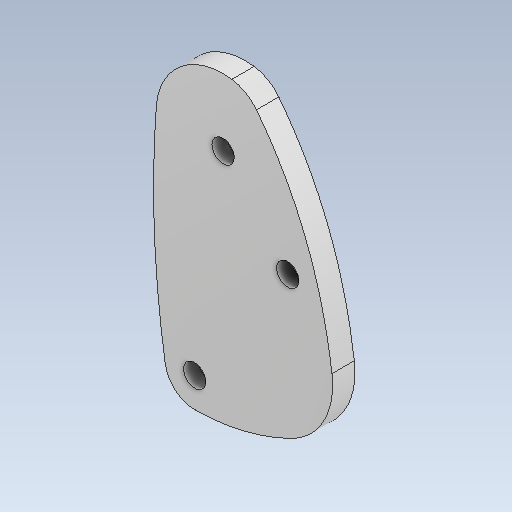
# Autodesk Inventor part: アンノーン後
Saved by Autodesk Inventor 2020.4 (Build 244396000, 396)
## iProperties
Created: 2021-02-23
Part Number: アンノーン後
Material: アルミニウム 2014-T4
Document SubType Name: Modeling
Designer: AA19065
Density: 2.8 g/cm^3
Appearance: サテン
Mass: 6.17685 g
Surface Area: 19.5398 cm^2
Volume: 2.20602 cm^3
Author: AA19065
Autodesk Inventor part; units mm, degrees
ref_plane "YZ Plane" through (0, 0, 0) normal (1, 0, 0) x (0, 1, 0)
ref_plane "XZ Plane" through (0, 0, 0) normal (0, 1, 0) x (-1, 0, 0)
ref_plane "XY Plane" through (0, 0, 0) normal (0, 0, 1) x (1, 0, 0)
sketch "スケッチ1" plane through (0, 0, 0) normal (0, 0, 1) x (1, 0, 0)
  line L0 (108, 72.831817) -> (108, -27.637331) construction
  circle A0 centre (90, 27) radius 3
  circle A1 centre (104.07345, 2) radius 6.025
  circle A2 centre (90, 27) radius 1.5
  circle A3 centre (104.07345, 2) radius 1.5
  circle A4 centre (82.04031, 11.281864) radius 1.5
  circle A5 centre (82.5, -8) radius 3
  circle A6 centre (82.5, -8) radius 1.5
  arc A7 (66.645247, -5.64) -> (72.915941, -4.36) centre (69.780594, -5) ccw
  arc A8 (72.724551, 23.828571) -> (66.645247, -5.64) centre (104.07345, 2) ccw
  arc A9 (77.976723, 20.171429) -> (72.915941, -4.36) centre (104.07345, 2) ccw
  arc A10 (77.976723, 20.171429) -> (72.724551, 23.828571) centre (75.350637, 22) ccw
  circle A11 centre (137.322151, 20) radius 1.25
  circle A12 centre (133.5, -8) radius 3
  circle A13 centre (133.5, -8) radius 1.5
  circle A14 centre (146, 10) radius 1.5
  arc A15 (-6.089587, 13.373015) -> (73.990447, 1.93301) centre (42.288654, 66.020578) ccw construction
  line L1 (108, 72.831817) -> (108, -27.637331) construction
  arc A16 (142.009553, 1.93301) -> (222.089587, 13.373015) centre (173.711346, 66.020578) ccw construction
  arc A17 (142.29705, -19.072921) -> (142.660887, 27.253552) centre (125.709293, 4.222021) ccw
  arc A18 (136.80781, 35.127338) -> (180.06622, 10.718677) centre (180.861669, 62.665248) ccw
  circle A19 centre (137.322151, 20) radius 9.006449
  arc A20 (128.322651, 20.353731) -> (130.555913, -8.5765) centre (253.226204, 15.444317) ccw
  arc A21 (133.414591, -10.998784) -> (152.948723, -4.485529) centre (134.268683, 18.989056) ccw
  arc A22 (35.93378, 10.718677) -> (79.19219, 35.127338) centre (35.138331, 62.665248) ccw
  arc A23 (73.339113, 27.253552) -> (73.70295, -19.072921) centre (90.290707, 4.222021) ccw
  arc A24 (90.887703, 29.865656) -> (71.118535, 25.188537) centre (84.969685, 10.761283) ccw
  arc A25 (109.559222, 4.491371) -> (92.075879, 29.165808) centre (36.719095, -28.589074) ccw
  arc A26 (80.567193, -10.294397) -> (70.653319, -16.566942) centre (76.603177, -15) ccw
  circle A27 centre (76.603177, -15) radius 5 construction
  circle A28 centre (94, -11) radius 1.5
  circle A29 centre (94, -11) radius 3
  arc A30 (103.111347, -3.947687) -> (84.657245, -10.084777) centre (99.757959, -24.678215) ccw
  line L2 (108, 72.831817) -> (108, -27.637331) construction
  circle A31 centre (90, 27) radius 3
  circle A32 centre (104.07345, 2) radius 6.025
  circle A33 centre (90, 27) radius 1.5
  circle A34 centre (104.07345, 2) radius 1.5
  circle A35 centre (82.04031, 11.281864) radius 1.5
  circle A36 centre (82.5, -8) radius 3
  circle A37 centre (82.5, -8) radius 1.5
  arc A38 (66.645247, -5.64) -> (72.915941, -4.36) centre (69.780594, -5) ccw
  arc A39 (72.724551, 23.828571) -> (66.645247, -5.64) centre (104.07345, 2) ccw
  arc A40 (77.976723, 20.171429) -> (72.915941, -4.36) centre (104.07345, 2) ccw
  arc A41 (77.976723, 20.171429) -> (72.724551, 23.828571) centre (75.350637, 22) ccw
  circle A42 centre (137.322151, 20) radius 1.25
  circle A43 centre (133.5, -8) radius 4
  circle A44 centre (133.5, -8) radius 1.5
  circle A45 centre (146, 10) radius 1.5
  arc A46 (-6.089587, 13.373015) -> (73.990447, 1.93301) centre (42.288654, 66.020578) ccw construction
  line L3 (108, 72.831817) -> (108, -27.637331) construction
  arc A47 (142.009553, 1.93301) -> (222.089587, 13.373015) centre (173.711346, 66.020578) ccw construction
  arc A48 (142.29705, -19.072921) -> (142.660887, 27.253552) centre (125.709293, 4.222021) ccw
  arc A49 (136.80781, 35.127338) -> (180.06622, 10.718677) centre (180.861669, 62.665248) ccw
  circle A50 centre (137.322151, 20) radius 9.006449
  arc A51 (128.342019, 20.688016) -> (129.550355, -8.632697) centre (252.976757, 11.139082) ccw
  arc A52 (133.563777, -11.999492) -> (152.948723, -4.485529) centre (133.08545, 17.996695) ccw
  arc A53 (35.93378, 10.718677) -> (79.19219, 35.127338) centre (35.138331, 62.665248) ccw
  arc A54 (73.339113, 27.253552) -> (73.70295, -19.072921) centre (90.290707, 4.222021) ccw
  arc A55 (90.887703, 29.865656) -> (71.118535, 25.188537) centre (84.969685, 10.761283) ccw
  arc A56 (109.559222, 4.491371) -> (92.075879, 29.165808) centre (36.719095, -28.589074) ccw
  arc A57 (80.567193, -10.294397) -> (70.653319, -16.566942) centre (76.603177, -15) ccw
  circle A58 centre (76.603177, -15) radius 5 construction
  circle A59 centre (94, -11) radius 1.5
  circle A60 centre (94, -11) radius 3
  arc A61 (103.111347, -3.947687) -> (84.657245, -10.084777) centre (99.757959, -24.678215) ccw
  circle A62 centre (137.322151, 20) radius 1.5
  point P0 (0, 0)
  point P1 (0, 0)
  point P2 (0, 0)
  point P3 (153.490711, -2.560367)
  point P4 (70.420594, -8.135347)
  point P5 (68.814065, 23.104865)
  point P6 (143.754929, 26.303609)
  point P7 (147.185935, 23.104865)
  point P8 (0, 0)
  point P9 (153.490711, -2.560367)
  point P10 (152.948723, -4.485529)
  dimension "d0" = 2
  dimension "d1" = 30
  dimension "d2" = 125
  dimension "d3" = 80
  dimension "d4" = 20
  dimension "d5" = 6
  dimension "d6" = 21
  dimension "d14" = 2
  dimension "d15" = 30
  dimension "d16" = 125
  dimension "d17" = 80
  dimension "d18" = 20
  dimension "d19" = 6
  dimension "d20" = 21
  dimension "d25" = 3
  constraints: 93 point on circle, 61 centre point, 20 tangent, 8 end point, 6 symmetric about line, 3 coincident, 1 vertical, 40 other
  measures "d0" distance of point (153.491, -2.56) A21.end
  measures "d1" radius of A21
  measures "d2" radius of A20
  measures "d3" radius of A25
  measures "d4" radius of A24
  measures "d5" diameter of A29
  measures "d6" radius of A30
  measures "d14" distance of point (153.491, -2.56) A52.end
  measures "d15" radius of A52
  measures "d16" radius of A51
  measures "d17" radius of A56
  measures "d18" radius of A55
  measures "d19" diameter of A60
  measures "d20" radius of A61
  measures "d25" diameter of A62
extrude "押し出し1" add sketch "スケッチ1" along normal blind 3 contours A12 | A12 A20 A43 A21 | A12 A21 A43 A20 | A43 A51 A19 A20 | A20 A19 A18 A17 A21 A43 | A21 A52 A43 | A19
fillet "フィレット1" radius 3 1 edges at (152.9487, -4.4855, 1.5)
fillet "フィレット2" radius 5 1 edges at (147.1859, 23.1049, 1.5)
sketch "スケッチ3" plane through (0, 0, 0) normal (0, 0, -1) x (-1, 0, 0)
  arc A0 (-146.917757, 23.334729) -> (-147.45257, 22.797215) centre (-143.650945, 19.549502) ccw
  arc A1 (-147.45257, 22.797215) -> (-153.216482, -3.598627) centre (-125.709293, 4.222021) ccw
  arc A2 (-152.246999, -5.086525) -> (-133.563777, -11.999492) centre (-133.08545, 17.996695) ccw
  arc A3 (-133.563777, -11.999492) -> (-129.550355, -8.632697) centre (-133.5, -8) ccw
  arc A4 (-129.550355, -8.632697) -> (-128.342019, 20.688016) centre (-252.976757, 11.139082) ccw
  arc A5 (-128.342019, 20.688016) -> (-143.754929, 26.303609) centre (-137.322151, 20) ccw
  arc A6 (-146.917757, 23.334729) -> (-143.754929, 26.303609) centre (-180.861669, 62.665248) ccw
  circle A7 centre (-133.5, -8) radius 1.5
  circle A8 centre (-146, 10) radius 1.5
  circle A9 centre (-137.322151, 20) radius 3.1
  circle A10 centre (-146, 10) radius 3.1
  circle A11 centre (-133.5, -8) radius 3.1
  arc A12 (-153.216482, -3.598627) -> (-152.246999, -5.086525) centre (-150.330844, -2.778203) ccw
  circle A13 centre (-137.322151, 20) radius 1.5
  point P0 (0, 0)
  dimension "d21" = 6.2
  dimension "d22" = 6.2
  dimension "d23" = 6.2
  constraints: 3 centre point, 2 coincident, 1 concentric
  measures "d21" diameter of A9
  measures "d22" diameter of A10
  measures "d23" diameter of A11
extrude "押し出し2" cut sketch "スケッチ3" against normal blind 1 contours A9 | A10 | A11
sketch "スケッチ4" plane through (0, 0, 3) normal (0, 0, 1) x (1, 0, 0)
  arc A0 (147.45257, 22.797215) -> (146.917757, 23.334729) centre (143.650945, 19.549502) ccw
  arc A1 (143.754929, 26.303609) -> (146.917757, 23.334729) centre (180.861669, 62.665248) ccw
  arc A2 (143.754929, 26.303609) -> (128.342019, 20.688016) centre (137.322151, 20) ccw
  arc A3 (128.342019, 20.688016) -> (129.550355, -8.632697) centre (252.976757, 11.139082) ccw
  arc A4 (129.550355, -8.632697) -> (133.563777, -11.999492) centre (133.5, -8) ccw
  arc A5 (133.563777, -11.999492) -> (152.246999, -5.086525) centre (133.08545, 17.996695) ccw
  arc A6 (152.246999, -5.086525) -> (153.216482, -3.598627) centre (150.330844, -2.778203) ccw
  arc A7 (153.216482, -3.598627) -> (147.45257, 22.797215) centre (125.709293, 4.222021) ccw
  circle A8 centre (146, 10) radius 1.5
  circle A9 centre (137.322151, 20) radius 1.5
  circle A10 centre (133.5, -8) radius 1.5
  arc A11 (153.216482, -3.598627) -> (147.45257, 22.797215) centre (125.709293, 4.222021) ccw
  arc A12 (143.754929, 26.303609) -> (128.342019, 20.688016) centre (137.322151, 20) ccw
  spline S0 degree 2 poles (140.758179, 28.325252) (151.754441, 15.122285) (152.532068, -5.69497) knots 0 0 0 1 1 1
  circle A13 centre (146, 10) radius 3.1
  point P0 (0, 0)
  point P1 (148.894459, 14.077022)
  point P2 (140.758179, 28.325252)
  point P3 (153.361481, -3.069376)
  point P4 (152.496355, -4.854392)
  dimension "d36" = 5
  dimension "d37" = 13
  dimension "d38" = 17
  dimension "d39" = 36
  constraints: 2 point on circle, 3 other
  measures "d36" distance of A8.centre point (148.894, 14.077)
  measures "d37" distance of A9.centre point (148.894, 14.077)
  measures "d38" distance of A8.centre point (152.532, -5.695)
  measures "d39" distance of point (152.532, -5.695) point (140.758, 28.325)
extrude "押し出し3" cut sketch "スケッチ4" against normal blind 10 contours A7 A6 S0 A2 A1 A0
fillet "フィレット3" radius 10 1 edges at (152.4964, -4.8544, 1.5)
fillet "フィレット4" radius 5 1 edges at (140.7582, 28.3253, 1.5)
